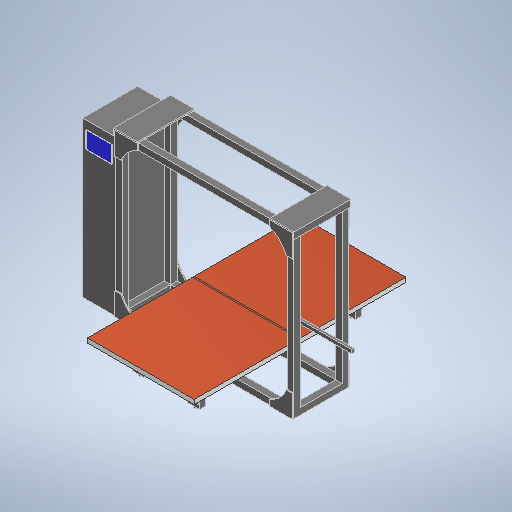
# Autodesk Inventor part: Lulzbot Taz 6
Saved by Autodesk Inventor 2025.2 (Build 292293000, 293)
## iProperties
Created: 2025-03-06
Part Number: Lulzbot Taz 6
Material: Generic
Document SubType Name: Modeling
Designer: Martinkowski
Density: 1 g/cm^3
Appearance: Default
Author: Martinkowski
Autodesk Inventor part; units mm, degrees
ref_plane "YZ Plane" through (0, 0, 0) normal (1, 0, 0) x (0, 1, 0)
ref_plane "XY Plane" through (0, 0, 0) normal (0, 0, 1) x (1, 0, 0)
sketch "Sketch5" plane through (0, 0, 0) normal (0, 0, 1) x (1, 0, 0)
  line L0 (0, 0) -> (102.631, 0)
  line L1 (102.631, 0) -> (102.631, 480)
  line L2 (102.631, 480) -> (0, 480)
  line L3 (0, 480) -> (0, 0)
  dimension "d12" = 102.631
  dimension "d13" = 480
  constraints: 8 end point, 2 parallel, 1 horizontal, 1 perpendicular
  measures "d12" distance of L1.end L2.end
  measures "d13" distance of L2.end L0.start
extrude "Extrusion5" add sketch "Sketch5" along normal mid plane 170
sketch "Sketch6" plane through (0, 0, 85) normal (0, 0, -1) x (1, 0, 0)
  line L0 (102.631, 0) -> (652.631, 0)
  line L1 (652.631, 0) -> (652.631, -500)
  line L2 (652.631, -500) -> (102.631, -500)
  line L3 (102.631, -500) -> (102.631, 0)
  line L4 (122.631, -480) -> (632.631, -480)
  line L5 (632.631, -480) -> (632.631, -20)
  line L6 (632.631, -20) -> (122.631, -20)
  line L7 (122.631, -20) -> (122.631, -480)
  dimension "d21" = 550
  dimension "d22" = 500
  dimension "d23" = 20
  constraints: 16 end point, 4 parallel, 2 perpendicular, 1 horizontal, 3 other
  measures "d21" distance of L1.end L2.end
  measures "d22" distance of L0.end L1.end
  measures "d23" distance between parallel lines of L4 L2
extrude "Extrusion6" add sketch "Sketch6" along normal blind 20 separate body
mirror "Mirror1" about plane through (0, 0, 0) normal (0, 0, 1) of "Extrusion6" bodies 2
sketch "Sketch7" plane through (0, 0, 0) normal (0, 0, 1) x (1, 0, 0)
  line L0 (102.631, 500) -> (652.631, 500) projected
  line L1 (632.631, 480) -> (122.631, 480) projected
  line L2 (102.631, 500) -> (122.631, 500)
  line L3 (122.631, 500) -> (122.631, 480)
  line L4 (122.631, 480) -> (102.631, 480)
  line L5 (102.631, 480) -> (102.631, 500)
  line L6 (652.631, 500) -> (652.631, 0) projected
  line L7 (632.631, 20) -> (652.631, 20)
  line L8 (652.631, 20) -> (652.631, 0)
  line L9 (652.631, 0) -> (632.631, 0)
  line L10 (632.631, 0) -> (632.631, 20)
  line L11 (632.631, 480) -> (652.631, 480)
  line L12 (652.631, 480) -> (652.631, 500)
  line L13 (652.631, 500) -> (632.631, 500)
  line L14 (632.631, 500) -> (632.631, 480)
  line L15 (122.631, 20) -> (102.631, 20)
  line L16 (102.631, 20) -> (102.631, 0)
  line L17 (102.631, 0) -> (122.631, 0)
  line L18 (122.631, 0) -> (122.631, 20)
  point P0 (0, 0)
  constraints: 32 end point, 8 parallel, 5 point on line, 4 horizontal, 4 perpendicular, 1 coincident
extrude "Extrusion7" add sketch "Sketch7" along normal mid plane 130 contours L0 L3 L4 L5 | L0 L6 L11 L14 | L6 L9 L10 L7 | L18 L17 L16 L15 bodies 2
ref_plane "Work Plane1" through (0, 0, 205) normal (0, 0, 1) x (1, 0, 0)
sketch "Sketch8" plane through (0, 0, 205) normal (0, 0, 1) x (1, 0, 0)
  line L0 (122.631, 20) -> (632.631, 20) projected
  line L1 (277.631, 20) -> (297.631, 20)
  line L2 (297.631, 20) -> (297.631, 40)
  line L3 (297.631, 40) -> (277.631, 40)
  line L4 (277.631, 40) -> (277.631, 20)
  line L5 (457.631, 20) -> (477.631, 20)
  line L6 (477.631, 20) -> (477.631, 40)
  line L7 (477.631, 40) -> (457.631, 40)
  line L8 (457.631, 40) -> (457.631, 20)
  line L9 (102.631, 0) -> (102.631, 480) projected
  point P0 (0, 0)
  dimension "d27" = 20
  dimension "d28" = 200
  dimension "d29" = 175
  constraints: 16 end point, 4 parallel, 3 equal length, 2 horizontal, 2 perpendicular, 2 point on line
  measures "d27" distance of L3.end L1.start
  measures "d28" distance between parallel lines of L6 L4
  measures "d29" distance between parallel lines of L4 L9
extrude "Extrusion8" add sketch "Sketch8" against normal blind 500 bodies 2
ref_plane "Work Plane2" through (0, 0, -45) normal (0, 0, 1) x (1, 0, 0)
sketch "Sketch9" plane through (0, 0, 205) normal (0, 0, 1) x (1, 0, 0)
  arc A0 (377.631, 70.1731) -> (273.381, 45.19) centre (377.631, -159.8269) ccw
  arc A1 (377.631, 29.0633) -> (305.881, 15.75) centre (377.631, -170.9367) ccw
  line L0 (305.881, 15.75) -> (273.381, 15.75)
  line L1 (273.381, 15.75) -> (273.381, 45.19)
  line L2 (377.631, 70.1731) -> (377.631, 29.0633)
  arc A2 (481.881, 45.19) -> (377.631, 70.1731) centre (377.631, -159.8269) ccw
  arc A3 (449.381, 15.75) -> (377.631, 29.0633) centre (377.631, -170.9367) ccw
  line L3 (449.381, 15.75) -> (481.881, 15.75)
  line L4 (481.881, 15.75) -> (481.881, 45.19)
  line L5 (277.631, 40) -> (277.631, 20) projected
  line L6 (277.631, 20) -> (297.631, 20) projected
  line L7 (297.631, 20) -> (297.631, 40) projected
  line L8 (297.631, 40) -> (277.631, 40) projected
  line L9 (457.631, 40) -> (457.631, 20) projected
  line L10 (457.631, 20) -> (477.631, 20) projected
  line L11 (477.631, 20) -> (477.631, 40) projected
  line L12 (477.631, 40) -> (457.631, 40) projected
  point P0 (0, 0)
  dimension "d34" = 4.25
  dimension "d35" = 4.25
  dimension "d36" = 200
  dimension "d37" = 4.25
  dimension "d39" = 8.25
  dimension "d40" = 29.44
  dimension "d41" = 230
  constraints: 10 end point, 8 point on circle, 5 symmetric about line, 4 centre point, 2 vertical, 1 concentric, 1 perpendicular, 1 vertical alignment, 2 other
  measures "d34" distance between parallel lines of L6 L0
  measures "d35" distance between parallel lines of L1 L5
  measures "d36" radius of A1
  measures "d37" distance between parallel lines of L4 L11
  measures "d39" distance from line of L0.start L7
  measures "d40" distance of L0.end L1.end
  measures "d41" radius of A0
extrude "Extrusion9" add sketch "Sketch9" along normal blind 4.763 separate body contours L2 A1 L0 L1 A0 | A2 L4 L3 A3 L2 | L8 L7 L6 L5 | L12 L11 L10 L9
mirror "Mirror2" about plane through (0, 0, -45) normal (0, 0, 1) of "Extrusion9" bodies 3
sketch "Sketch10" plane through (0, 0, 205) normal (0, 0, 1) x (1, 0, 0)
  line L0 (482.131, 0) -> (444.851, 0)
  line L1 (444.851, 0) -> (444.851, 77.78)
  line L2 (444.851, 77.78) -> (482.131, 77.78)
  line L3 (482.131, 77.78) -> (482.131, 0)
  line L4 (457.631, 40) -> (457.631, 20) projected
  line L5 (457.631, 20) -> (477.631, 20) projected
  line L6 (477.631, 20) -> (477.631, 40) projected
  line L7 (477.631, 40) -> (457.631, 40) projected
  circle A0 centre (452.631, 69.75) radius 5
  line L8 (652.631, 0) -> (102.631, 0) projected
  point P0 (0, 0)
  dimension "d42" = 77.78
  dimension "d44" = 4.5
  dimension "d45" = 37.28
  dimension "d46" = 10
  dimension "d47" = 25
  dimension "d48" = 49.75
  constraints: 8 end point, 2 parallel, 1 centre point, 1 collinear, 1 horizontal, 1 perpendicular
  measures "d42" distance of L2.end L0.start
  measures "d44" distance between parallel lines of L6 L3
  measures "d45" distance of L0.start L0.end
  measures "d46" diameter of A0
  measures "d47" distance from line of A0.centre L6
  measures "d48" distance from line of A0.centre L5
extrude "Extrusion10" add sketch "Sketch10" against normal blind 18 separate body
ref_plane "Work Plane3" through (377.631, 20, 205) normal (1, 0, 0) x (0, 0, -1)
mirror "Mirror3" about plane through (377.631, 20, 205) normal (1, 0, 0) bodies 4
mirror "Mirror4" about plane through (0, 0, -45) normal (0, 0, 1) bodies 4
sketch "Sketch11" plane through (0, 0, 205) normal (0, 0, 1) x (1, 0, 0)
  circle A0 centre (302.631, 69.75) radius 5 projected
  circle A1 centre (452.631, 69.75) radius 5 projected
  point P0 (0, 0)
extrude "Extrusion11" add sketch "Sketch11" against normal up to surface (500 mm away) separate body
sketch "Sketch12" plane through (0, 0, 0) normal (0, 0, 1) x (1, 0, 0)
  line L0 (102.631, 500) -> (652.631, 500) projected
  line L1 (582.631, 500) -> (656.631, 500)
  line L2 (656.631, 500) -> (656.631, 504)
  line L3 (656.631, 504) -> (582.631, 504)
  line L4 (582.631, 504) -> (582.631, 500)
  line L5 (652.631, 500) -> (652.631, 0) projected
  line L6 (652.631, 484) -> (656.631, 484)
  line L7 (656.631, 484) -> (656.631, 500)
  line L8 (656.631, 500) -> (652.631, 500)
  line L9 (652.631, 500) -> (652.631, 484)
  line L10 (377.631, 500) -> (377.631, 480)
  line L11 (632.631, 480) -> (122.631, 480) projected
  line L12 (172.631, 500) -> (98.631, 500)
  line L13 (98.631, 500) -> (98.631, 504)
  line L14 (98.631, 504) -> (172.631, 504)
  line L15 (172.631, 504) -> (172.631, 500)
  line L16 (102.631, 484) -> (98.631, 484)
  line L17 (98.631, 484) -> (98.631, 500)
  line L18 (98.631, 500) -> (102.631, 500)
  line L19 (102.631, 500) -> (102.631, 484)
  point P0 (0, 0)
  dimension "d53" = 4
  dimension "d54" = 74
  dimension "d55" = 20
  constraints: 34 end point, 8 symmetric about line, 4 parallel, 3 perpendicular, 2 horizontal, 2 midpoint, 2 point on line
  measures "d53" distance of L6.start L6.end
  measures "d54" distance of L2.end L3.end
  measures "d55" distance between parallel lines of L6 L3
extrude "Extrusion12" add sketch "Sketch12" along normal mid plane 176.35 separate body
sketch "Sketch13" plane through (0, 0, 88.175) normal (0, 0, 1) x (1, 0, 0)
  line L0 (582.631, 500) -> (652.631, 500) projected
  line L1 (652.631, 500) -> (652.631, 484) projected
  line L2 (102.631, 500) -> (652.631, 500) projected
  line L3 (377.631, 500) -> (377.631, 480)
  line L4 (632.631, 480) -> (122.631, 480) projected
  line L5 (632.631, 20) -> (632.631, 480) projected
  line L6 (632.631, 430) -> (652.631, 430)
  line L7 (652.631, 430) -> (652.631, 500)
  line L8 (652.631, 500) -> (632.631, 500)
  line L9 (632.631, 500) -> (632.631, 430)
  line L10 (632.631, 480) -> (652.631, 480) projected
  line L11 (582.631, 500) -> (652.631, 500)
  line L12 (652.631, 500) -> (652.631, 480)
  line L13 (652.631, 480) -> (582.631, 480)
  line L14 (582.631, 480) -> (582.631, 500)
  arc A0 (632.631, 430) -> (582.631, 480) centre (552.973, 400.342) ccw
  line L15 (172.631, 500) -> (102.631, 500)
  line L16 (102.631, 500) -> (102.631, 484)
  line L17 (122.631, 430) -> (102.631, 430)
  line L18 (102.631, 430) -> (102.631, 500)
  line L19 (102.631, 500) -> (122.631, 500)
  line L20 (122.631, 500) -> (122.631, 430)
  line L21 (122.631, 480) -> (102.631, 480)
  line L22 (172.631, 500) -> (102.631, 500)
  line L23 (102.631, 500) -> (102.631, 480)
  line L24 (102.631, 480) -> (172.631, 480)
  line L25 (172.631, 480) -> (172.631, 500)
  arc A1 (172.631, 480) -> (122.631, 430) centre (202.289, 400.342) ccw
  point P0 (0, 0)
  dimension "d58" = 70
  dimension "d59" = 85
  constraints: 40 end point, 11 symmetric about line, 4 parallel, 4 point on circle, 3 perpendicular, 2 centre point, 2 horizontal, 2 midpoint, 2 point on line, 1 other
  measures "d58" distance of L6.end L0.end
  measures "d59" radius of A0
extrude "Extrusion13" add sketch "Sketch13" against normal up to surface (3.175 mm away) separate body contours L0 L9 L4 L14 | L0 L1 L7 L10 L9 | L4 L5 A0 | L10 L7 L6 L5 | L25 L4 L20 L2 | L20 L21 L18 L16 L2 | A1 L20 L4 | L20 L17 L18 L21
ref_plane "Work Plane4" through (102.631, 250, 85) normal (0, 1, 0) x (1, 0, 0)
mirror "Mirror5" about plane through (102.631, 250, 85) normal (0, 1, 0) bodies 7
mirror "Mirror6" about plane through (0, 0, 0) normal (0, 0, 1) bodies 7
ref_plane "Work Plane5" through (0, 82.26, 0) normal (0, 1, 0) x (-1, 0, 0)
sketch "Sketch14" plane through (0, 82.26, 0) normal (0, 1, 0) x (-1, 0, 0)
  line L0 (-542.631, -372.5) -> (-212.631, -372.5)
  line L1 (-212.631, -372.5) -> (-212.631, -42.5)
  line L2 (-212.631, -42.5) -> (-542.631, -42.5)
  line L3 (-542.631, -42.5) -> (-542.631, -372.5)
  line L4 (-542.631, -372.5) -> (-212.631, -42.5) construction
  line L5 (-212.631, -372.5) -> (-542.631, -42.5) construction
  line L6 (-377.631, -726.3127) -> (-377.631, 365.7756) projected
  line L7 (-477.801, -241) -> (-427.461, -241)
  line L8 (-427.461, -241) -> (-427.461, -277)
  line L9 (-427.461, -277) -> (-477.801, -277)
  line L10 (-477.801, -277) -> (-477.801, -241)
  line L11 (-477.801, -241) -> (-427.461, -277) construction
  line L12 (-427.461, -241) -> (-477.801, -277) construction
  line L13 (-457.631, 205) -> (-457.631, -295) projected
  line L14 (-447.631, 205) -> (-447.631, -295) projected
  line L15 (-457.631, -200.0911) -> (-447.631, -200.0911) construction
  line L16 (-452.631, -217.6251) -> (-452.631, -182.5571)
  line L17 (-420.0518, -207.5) -> (-335.2102, -207.5) construction
  line L18 (-477.801, -174) -> (-427.461, -174)
  line L19 (-427.461, -174) -> (-427.461, -138)
  line L20 (-427.461, -138) -> (-477.801, -138)
  line L21 (-477.801, -138) -> (-477.801, -174)
  line L22 (-477.801, -174) -> (-427.461, -138) construction
  line L23 (-427.461, -174) -> (-477.801, -138) construction
  line L24 (-444.851, -277) -> (-482.131, -277) projected
  point P0 (0, 0)
  point P1 (-377.631, -207.5)
  point P2 (-452.631, -259)
  point P3 (-452.631, -200.0911)
  point P4 (-452.631, -156)
  point P5 (-452.631, -197.3749)
  dimension "d63" = 330
  dimension "d64" = 95.5
  dimension "d65" = 36
  dimension "d66" = 50.34
  dimension "d67" = 0
  constraints: 42 end point, 7 midpoint, 6 symmetric about line, 4 parallel, 4 perpendicular, 4 point on line, 3 horizontal, 1 vertical
  measures "d63" distance of L0.start L0.end
  measures "d64" distance between parallel lines of L9 L0
  measures "d65" distance of L7.end L8.end
  measures "d66" distance of L8.end L9.end
  measures "d67" distance between parallel lines of L24 L9
extrude "Extrusion14" add sketch "Sketch14" along normal blind 13.75 separate body
mirror "Mirror7" about plane through (0, 0, -45) normal (0, 0, 1) bodies 8 separate body
sketch "Sketch15" plane through (0, 0, 0) normal (0, 1, 0) x (-1, 0, 0)
  circle A0 centre (-32.03, 35) radius 6.5
  circle A1 centre (-291.591, 196) radius 6.5
  circle A2 centre (-129.131, 75) radius 6.5
  line L0 (0, -85) -> (0, 85) projected
  line L1 (0, 85) -> (-102.631, 85) projected
  line L2 (-122.631, -65) -> (-122.631, 65) projected
  line L3 (-122.631, 85) -> (-122.631, 65) projected
  line L4 (-122.631, 65) -> (-122.631, 85)
  line L5 (-310.411, 205) -> (-310.411, 187) projected
  line L6 (-102.631, 85) -> (-102.631, -85) projected
  line L7 (-273.131, 205) -> (-273.131, 187) projected
  line L8 (-297.631, 65) -> (-457.631, 65) projected
  line L9 (-377.631, 65) -> (-377.631, -174.6881)
  line L10 (-122.631, 0) -> (-558.5477, 0)
  circle A3 centre (-129.131, -75) radius 6.5
  circle A4 centre (-626.131, 75) radius 6.5
  circle A5 centre (-626.131, -75) radius 6.5
  line L11 (-449.381, 205) -> (-305.881, 205) projected
  line L12 (-377.631, 205) -> (-377.631, 126.4005)
  line L13 (-297.631, 205) -> (-297.631, -295) projected
  line L14 (-297.631, -45) -> (-569.3906, -45)
  line L15 (-212.631, -42.5) -> (-542.631, -42.5) projected
  circle A6 centre (-291.591, -286) radius 6.5
  circle A7 centre (-463.671, 196) radius 6.5
  circle A8 centre (-463.671, -286) radius 6.5
  point P0 (0, 0)
  point P1 (-122.631, 75)
  point P2 (-310.411, 196)
  point P3 (-297.631, 198.4017)
  point P4 (-297.631, 193.5983)
  dimension "d70" = 13
  dimension "d71" = 32.03
  dimension "d72" = 50
  dimension "d73" = 26.5
  dimension "d74" = 18.46
  constraints: 10 end point, 9 centre point, 6 midpoint, 6 symmetric about line, 3 vertical, 2 equal radius, 2 horizontal alignment, 1 horizontal, 1 parallel, 6 other
  measures "d70" diameter of A0
  measures "d71" distance from line of A0.centre L0
  measures "d72" distance from line of A0.centre L1
  measures "d73" distance from line of A2.centre L6
  measures "d74" distance from line of A1.centre L7
extrude "Extrusion15" add sketch "Sketch15" against normal blind 7 separate body contours A0 | A1 L13 | A2 | A3 | A4 | A5 | A6 L13 | L13 A6 | A7 | A8 picked at (-293.7821, 195.1994)
sketch "Sketch16" plane through (0, 0, 85) normal (0, 0, 1) x (1, 0, 0)
  line L0 (102.631, 480) -> (0, 480) projected
  line L1 (11.3155, 401.95) -> (91.3155, 401.95)
  line L2 (91.3155, 401.95) -> (91.3155, 454.95)
  line L3 (91.3155, 454.95) -> (11.3155, 454.95)
  line L4 (11.3155, 454.95) -> (11.3155, 401.95)
  line L5 (11.3155, 401.95) -> (91.3155, 454.95) construction
  line L6 (91.3155, 401.95) -> (11.3155, 454.95) construction
  point P0 (51.3155, 428.45)
  point P1 (51.3155, 480)
  dimension "d77" = 80
  dimension "d78" = 53
  dimension "d79" = 25.05
  constraints: 12 end point, 3 midpoint, 2 parallel, 1 horizontal, 1 perpendicular, 1 vertical alignment
  measures "d77" distance of L2.end L3.end
  measures "d78" distance of L3.end L1.start
  measures "d79" distance between parallel lines of L3 L0
extrude "Extrusion16" add sketch "Sketch16" along normal blind 1 bodies 1
sketch "Sketch17" plane through (0, 0, 65) normal (0, 0, -1) x (-1, 0, 0)
  line L0 (-652.631, 480) -> (-652.631, 20) projected
  line L1 (-632.631, 20) -> (-632.631, 480) projected
  line L2 (-632.631, 255.58) -> (-812.631, 255.58)
  line L3 (-812.631, 255.58) -> (-812.631, 244.15)
  line L4 (-812.631, 244.15) -> (-632.631, 244.15)
  line L5 (-632.631, 244.15) -> (-632.631, 255.58)
  line L6 (-975.1572, 0) -> (162.5262, 0) projected
  point P0 (0, 0)
  point P1 (-652.631, 244.15)
  point P2 (-652.631, 255.58)
  dimension "d82" = 160
  dimension "d83" = 11.43
  dimension "d84" = 255.58
  constraints: 8 end point, 2 parallel, 1 horizontal, 1 perpendicular, 1 point on line
  measures "d82" distance from line of L3.end L0
  measures "d83" distance between parallel lines of L4 L2
  measures "d84" distance between parallel lines of L2 L6
extrude "Extrusion17" add sketch "Sketch17" along normal blind 7.5 bodies 2
equation "\"d37\" = d34"
body "Solid2"
body "Solid3"
body "Solid5"
body "Solid6"
body "Solid7"
body "Solid8"
body "Solid9"
body "Solid10"
body "Solid11"
body "Solid12"
